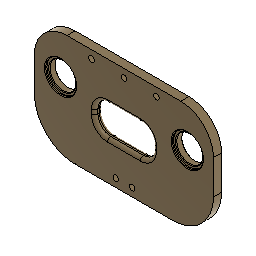
Outer Plate (Autodesk Fusion 360 design; units mm, degrees)
Autodesk Fusion 360 part; units mm, degrees
sketch "Sketch1" plane through (0, 58.6943, 0) normal (0, 1, 0) x (-1, 0, 0)
  line L0 (-161.4765, 498.7395) -> (-162.948, 497.802)
  line L1 (-162.948, 497.802) -> (-164.3322, 496.7399)
  line L2 (-164.3322, 496.7399) -> (-165.6186, 495.5611)
  line L3 (-165.6186, 495.5611) -> (-166.7974, 494.2748)
  line L4 (-166.7974, 494.2748) -> (-167.8595, 492.8905)
  line L5 (-167.8595, 492.8905) -> (-168.797, 491.419)
  line L6 (-168.797, 491.419) -> (-169.6026, 489.8714)
  line L7 (-169.6026, 489.8714) -> (-170.2703, 488.2594)
  line L8 (-170.2703, 488.2594) -> (-170.795, 486.5954)
  line L9 (-170.795, 486.5954) -> (-171.1726, 484.892)
  line L10 (-171.1726, 484.892) -> (-171.4004, 483.1621)
  line L11 (-171.4004, 483.1621) -> (-171.4765, 481.419)
  line L12 (-171.4765, 481.419) -> (-171.4765, 460.419)
  line L13 (-171.4765, 460.419) -> (-171.3994, 458.4576)
  line L14 (-171.3994, 458.4576) -> (-171.1687, 456.5082)
  line L15 (-171.1687, 456.5082) -> (-170.7857, 454.5829)
  line L16 (-170.7857, 454.5829) -> (-170.2529, 452.6936)
  line L17 (-170.2529, 452.6936) -> (-169.5735, 450.8519)
  line L18 (-169.5735, 450.8519) -> (-168.7516, 449.0692)
  line L19 (-168.7516, 449.0692) -> (-167.7925, 447.3565)
  line L20 (-167.7925, 447.3565) -> (-166.7019, 445.7244)
  line L21 (-166.7019, 445.7244) -> (-165.4866, 444.1828)
  line L22 (-165.4866, 444.1828) -> (-164.1541, 442.7413)
  line L23 (-164.1541, 442.7413) -> (-162.7127, 441.4089)
  line L24 (-162.7127, 441.4089) -> (-161.1711, 440.1936)
  line L25 (-161.1711, 440.1936) -> (-159.5389, 439.103)
  line L26 (-159.5389, 439.103) -> (-157.8262, 438.1439)
  line L27 (-157.8262, 438.1439) -> (-156.0436, 437.322)
  line L28 (-156.0436, 437.322) -> (-154.2019, 436.6426)
  line L29 (-154.2019, 436.6426) -> (-152.3126, 436.1098)
  line L30 (-152.3126, 436.1098) -> (-150.3873, 435.7268)
  line L31 (-150.3873, 435.7268) -> (-148.4379, 435.4961)
  line L32 (-148.4379, 435.4961) -> (-146.4765, 435.419)
  line L33 (-146.4765, 435.419) -> (-86.4765, 435.419)
  line L34 (-86.4765, 435.419) -> (-84.515, 435.4961)
  line L35 (-84.515, 435.4961) -> (-82.5656, 435.7268)
  line L36 (-82.5656, 435.7268) -> (-80.6403, 436.1098)
  line L37 (-80.6403, 436.1098) -> (-78.751, 436.6426)
  line L38 (-78.751, 436.6426) -> (-76.9094, 437.322)
  line L39 (-76.9094, 437.322) -> (-75.1267, 438.1439)
  line L40 (-75.1267, 438.1439) -> (-73.414, 439.103)
  line L41 (-73.414, 439.103) -> (-71.7818, 440.1936)
  line L42 (-71.7818, 440.1936) -> (-70.2403, 441.4089)
  line L43 (-70.2403, 441.4089) -> (-68.7988, 442.7413)
  line L44 (-68.7988, 442.7413) -> (-67.4663, 444.1828)
  line L45 (-67.4663, 444.1828) -> (-66.251, 445.7244)
  line L46 (-66.251, 445.7244) -> (-65.1605, 447.3565)
  line L47 (-65.1605, 447.3565) -> (-64.2013, 449.0692)
  line L48 (-64.2013, 449.0692) -> (-63.3795, 450.8519)
  line L49 (-63.3795, 450.8519) -> (-62.7, 452.6936)
  line L50 (-62.7, 452.6936) -> (-62.1672, 454.5829)
  line L51 (-62.1672, 454.5829) -> (-61.7843, 456.5082)
  line L52 (-61.7843, 456.5082) -> (-61.5535, 458.4576)
  line L53 (-61.5535, 458.4576) -> (-61.4765, 460.419)
  line L54 (-61.4765, 460.419) -> (-61.4765, 481.419)
  line L55 (-61.4765, 481.419) -> (-61.5526, 483.1621)
  line L56 (-61.5526, 483.1621) -> (-61.7803, 484.892)
  line L57 (-61.7803, 484.892) -> (-62.1579, 486.5954)
  line L58 (-62.1579, 486.5954) -> (-62.6826, 488.2594)
  line L59 (-62.6826, 488.2594) -> (-63.3503, 489.8714)
  line L60 (-63.3503, 489.8714) -> (-64.1559, 491.419)
  line L61 (-64.1559, 491.419) -> (-65.0934, 492.8905)
  line L62 (-65.0934, 492.8905) -> (-66.1556, 494.2748)
  line L63 (-66.1556, 494.2748) -> (-67.3343, 495.5611)
  line L64 (-67.3343, 495.5611) -> (-68.6207, 496.7399)
  line L65 (-68.6207, 496.7399) -> (-70.0049, 497.802)
  line L66 (-70.0049, 497.802) -> (-71.4765, 498.7395)
  line L67 (-71.4765, 498.7395) -> (-73.0241, 499.5452)
  line L68 (-73.0241, 499.5452) -> (-74.6361, 500.2129)
  line L69 (-74.6361, 500.2129) -> (-76.3001, 500.7375)
  line L70 (-76.3001, 500.7375) -> (-78.0035, 501.1151)
  line L71 (-78.0035, 501.1151) -> (-79.7333, 501.3429)
  line L72 (-79.7333, 501.3429) -> (-81.4765, 501.419)
  line L73 (-81.4765, 501.419) -> (-151.4765, 501.419)
  line L74 (-151.4765, 501.419) -> (-153.2196, 501.3429)
  line L75 (-153.2196, 501.3429) -> (-154.9494, 501.1151)
  line L76 (-154.9494, 501.1151) -> (-156.6528, 500.7375)
  line L77 (-156.6528, 500.7375) -> (-158.3169, 500.2129)
  line L78 (-158.3169, 500.2129) -> (-159.9288, 499.5452)
  line L79 (-159.9288, 499.5452) -> (-161.4765, 498.7395)
  line L80 (-124.4561, 440.0705) -> (-124.4561, 440.767)
  line L81 (-124.4561, 440.767) -> (-124.2954, 441.4448)
  line L82 (-124.2954, 441.4448) -> (-123.9828, 442.0672)
  line L83 (-123.9828, 442.0672) -> (-123.5351, 442.6007)
  line L84 (-123.5351, 442.6007) -> (-122.9765, 443.0167)
  line L85 (-122.9765, 443.0167) -> (-122.3369, 443.2925)
  line L86 (-122.3369, 443.2925) -> (-121.651, 443.4135)
  line L87 (-121.651, 443.4135) -> (-120.9557, 443.373)
  line L88 (-120.9557, 443.373) -> (-120.2884, 443.1732)
  line L89 (-120.2884, 443.1732) -> (-119.6852, 442.825)
  line L90 (-119.6852, 442.825) -> (-119.1786, 442.347)
  line L91 (-119.1786, 442.347) -> (-118.7959, 441.7651)
  line L92 (-118.7959, 441.7651) -> (-118.5577, 441.1106)
  line L93 (-118.5577, 441.1106) -> (-118.4768, 440.4188)
  line L94 (-118.4768, 440.4188) -> (-118.5577, 439.727)
  line L95 (-118.5577, 439.727) -> (-118.7959, 439.0725)
  line L96 (-118.7959, 439.0725) -> (-119.1786, 438.4906)
  line L97 (-119.1786, 438.4906) -> (-119.6852, 438.0126)
  line L98 (-119.6852, 438.0126) -> (-120.2884, 437.6643)
  line L99 (-120.2884, 437.6643) -> (-120.9557, 437.4646)
  line L100 (-120.9557, 437.4646) -> (-121.651, 437.4241)
  line L101 (-121.651, 437.4241) -> (-122.3369, 437.545)
  line L102 (-122.3369, 437.545) -> (-122.9765, 437.8209)
  line L103 (-122.9765, 437.8209) -> (-123.5351, 438.2369)
  line L104 (-123.5351, 438.2369) -> (-123.9828, 438.7704)
  line L105 (-123.9828, 438.7704) -> (-124.2954, 439.3928)
  line L106 (-124.2954, 439.3928) -> (-124.4561, 440.0705)
  line L107 (-90.9566, 487.2028) -> (-90.3766, 487.4647)
  line L108 (-90.3766, 487.4647) -> (-89.75, 487.5755)
  line L109 (-89.75, 487.5755) -> (-89.1154, 487.5283)
  line L110 (-89.1154, 487.5283) -> (-88.5121, 487.326)
  line L111 (-88.5121, 487.326) -> (-83.3137, 484.827)
  line L112 (-83.3137, 484.827) -> (-82.2929, 493.5729)
  line L113 (-82.2929, 493.5729) -> (-82.1336, 493.5729)
  line L114 (-82.1336, 493.5729) -> (-82.0349, 494.419)
  line L115 (-82.0349, 494.419) -> (-80.1169, 494.419)
  line L116 (-80.1169, 494.419) -> (-80.1158, 494.4247)
  line L117 (-80.1158, 494.4247) -> (-79.9215, 495.053)
  line L118 (-79.9215, 495.053) -> (-79.5884, 495.6199)
  line L119 (-79.5884, 495.6199) -> (-79.1342, 496.0954)
  line L120 (-79.1342, 496.0954) -> (-78.5831, 496.4542)
  line L121 (-78.5831, 496.4542) -> (-77.9645, 496.6771)
  line L122 (-77.9645, 496.6771) -> (-77.3112, 496.7523)
  line L123 (-77.3112, 496.7523) -> (-76.6581, 496.6758)
  line L124 (-76.6581, 496.6758) -> (-76.04, 496.4516)
  line L125 (-76.04, 496.4516) -> (-75.4896, 496.0917)
  line L126 (-75.4896, 496.0917) -> (-75.0364, 495.6152)
  line L127 (-75.0364, 495.6152) -> (-74.7044, 495.0476)
  line L128 (-74.7044, 495.0476) -> (-74.5114, 494.419)
  line L129 (-74.5114, 494.419) -> (-73.034, 494.419)
  line L130 (-73.034, 494.419) -> (-72.9352, 493.5729)
  line L131 (-72.9352, 493.5729) -> (-72.6609, 493.5729)
  line L132 (-72.6609, 493.5729) -> (-71.6401, 484.8274)
  line L133 (-71.6401, 484.8274) -> (-66.4424, 487.326)
  line L134 (-66.4424, 487.326) -> (-65.8391, 487.5283)
  line L135 (-65.8391, 487.5283) -> (-65.2045, 487.5755)
  line L136 (-65.2045, 487.5755) -> (-64.5779, 487.4647)
  line L137 (-64.5779, 487.4647) -> (-63.9979, 487.2028)
  line L138 (-63.9979, 487.2028) -> (-63.5005, 486.806)
  line L139 (-63.5005, 486.806) -> (-63.1163, 486.2987)
  line L140 (-63.1163, 486.2987) -> (-62.5715, 485.355)
  line L141 (-62.5715, 485.355) -> (-62.3346, 484.8044)
  line L142 (-62.3346, 484.8044) -> (-62.2323, 484.2138)
  line L143 (-62.2323, 484.2138) -> (-62.2701, 483.6156)
  line L144 (-62.2701, 483.6156) -> (-62.4459, 483.0425)
  line L145 (-62.4459, 483.0425) -> (-62.7502, 482.5261)
  line L146 (-62.7502, 482.5261) -> (-63.1661, 482.0945)
  line L147 (-63.1661, 482.0945) -> (-68.93, 477.3722)
  line L148 (-68.93, 477.3722) -> (-63.1661, 472.6498)
  line L149 (-63.1661, 472.6498) -> (-62.7502, 472.2182)
  line L150 (-62.7502, 472.2182) -> (-62.4459, 471.7018)
  line L151 (-62.4459, 471.7018) -> (-62.2701, 471.1287)
  line L152 (-62.2701, 471.1287) -> (-62.2323, 470.5305)
  line L153 (-62.2323, 470.5305) -> (-62.3346, 469.9399)
  line L154 (-62.3346, 469.9399) -> (-62.5715, 469.3893)
  line L155 (-62.5715, 469.3893) -> (-63.1163, 468.4456)
  line L156 (-63.1163, 468.4456) -> (-63.5005, 467.9383)
  line L157 (-63.5005, 467.9383) -> (-63.9979, 467.5415)
  line L158 (-63.9979, 467.5415) -> (-64.5779, 467.2796)
  line L159 (-64.5779, 467.2796) -> (-65.2045, 467.1688)
  line L160 (-65.2045, 467.1688) -> (-65.8391, 467.216)
  line L161 (-65.8391, 467.216) -> (-66.4424, 467.4183)
  line L162 (-66.4424, 467.4183) -> (-71.6506, 469.922)
  line L163 (-71.6506, 469.922) -> (-73.8018, 451.4907)
  line L164 (-73.8018, 451.4907) -> (-73.9694, 450.7417)
  line L165 (-73.9694, 450.7417) -> (-74.2878, 450.0434)
  line L166 (-74.2878, 450.0434) -> (-74.7435, 449.4259)
  line L167 (-74.7435, 449.4259) -> (-75.3168, 448.9156)
  line L168 (-75.3168, 448.9156) -> (-75.983, 448.5346)
  line L169 (-75.983, 448.5346) -> (-76.7135, 448.2992)
  line L170 (-76.7135, 448.2992) -> (-77.4769, 448.2196)
  line L171 (-77.4769, 448.2196) -> (-78.2402, 448.2992)
  line L172 (-78.2402, 448.2992) -> (-78.9707, 448.5346)
  line L173 (-78.9707, 448.5346) -> (-79.6369, 448.9156)
  line L174 (-79.6369, 448.9156) -> (-80.2102, 449.4259)
  line L175 (-80.2102, 449.4259) -> (-80.6659, 450.0434)
  line L176 (-80.6659, 450.0434) -> (-80.9844, 450.7417)
  line L177 (-80.9844, 450.7417) -> (-81.1519, 451.4907)
  line L178 (-81.1519, 451.4907) -> (-83.3277, 470.1324)
  line L179 (-83.3277, 470.1324) -> (-88.5987, 467.5986)
  line L180 (-88.5987, 467.5986) -> (-89.1549, 467.4121)
  line L181 (-89.1549, 467.4121) -> (-89.7399, 467.3686)
  line L182 (-89.7399, 467.3686) -> (-90.3176, 467.4707)
  line L183 (-90.3176, 467.4707) -> (-90.8523, 467.7121)
  line L184 (-90.8523, 467.7121) -> (-91.3108, 468.078)
  line L185 (-91.3108, 468.078) -> (-91.665, 468.5456)
  line L186 (-91.665, 468.5456) -> (-92.2102, 469.49)
  line L187 (-92.2102, 469.49) -> (-92.4286, 469.9976)
  line L188 (-92.4286, 469.9976) -> (-92.5229, 470.5421)
  line L189 (-92.5229, 470.5421) -> (-92.4881, 471.0935)
  line L190 (-92.4881, 471.0935) -> (-92.326, 471.6218)
  line L191 (-92.326, 471.6218) -> (-92.0455, 472.0979)
  line L192 (-92.0455, 472.0979) -> (-91.662, 472.4957)
  line L193 (-91.662, 472.4957) -> (-85.8673, 477.2434)
  line L194 (-85.8673, 477.2434) -> (-91.7884, 482.0945)
  line L195 (-91.7884, 482.0945) -> (-92.2044, 482.5261)
  line L196 (-92.2044, 482.5261) -> (-92.5086, 483.0425)
  line L197 (-92.5086, 483.0425) -> (-92.6845, 483.6156)
  line L198 (-92.6845, 483.6156) -> (-92.7222, 484.2138)
  line L199 (-92.7222, 484.2138) -> (-92.6199, 484.8044)
  line L200 (-92.6199, 484.8044) -> (-92.383, 485.355)
  line L201 (-92.383, 485.355) -> (-91.8382, 486.2987)
  line L202 (-91.8382, 486.2987) -> (-91.454, 486.806)
  line L203 (-91.454, 486.806) -> (-90.9566, 487.2028)
  line L204 (-97.3367, 499.2923) -> (-96.6509, 499.4133)
  line L205 (-96.6509, 499.4133) -> (-95.9555, 499.3728)
  line L206 (-95.9555, 499.3728) -> (-95.2883, 499.173)
  line L207 (-95.2883, 499.173) -> (-94.6852, 498.8248)
  line L208 (-94.6852, 498.8248) -> (-94.1785, 498.3468)
  line L209 (-94.1785, 498.3468) -> (-93.7958, 497.7649)
  line L210 (-93.7958, 497.7649) -> (-93.5576, 497.1104)
  line L211 (-93.5576, 497.1104) -> (-93.4768, 496.4187)
  line L212 (-93.4768, 496.4187) -> (-93.5576, 495.7269)
  line L213 (-93.5576, 495.7269) -> (-93.7958, 495.0724)
  line L214 (-93.7958, 495.0724) -> (-94.1785, 494.4905)
  line L215 (-94.1785, 494.4905) -> (-94.6852, 494.0126)
  line L216 (-94.6852, 494.0126) -> (-95.2883, 493.6643)
  line L217 (-95.2883, 493.6643) -> (-95.9555, 493.4646)
  line L218 (-95.9555, 493.4646) -> (-96.6509, 493.4241)
  line L219 (-96.6509, 493.4241) -> (-97.3367, 493.545)
  line L220 (-97.3367, 493.545) -> (-97.9763, 493.8209)
  line L221 (-97.9763, 493.8209) -> (-98.5349, 494.2368)
  line L222 (-98.5349, 494.2368) -> (-98.9826, 494.7703)
  line L223 (-98.9826, 494.7703) -> (-99.2952, 495.3927)
  line L224 (-99.2952, 495.3927) -> (-99.4558, 496.0704)
  line L225 (-99.4558, 496.0704) -> (-99.4558, 496.7669)
  line L226 (-99.4558, 496.7669) -> (-99.2952, 497.4446)
  line L227 (-99.2952, 497.4446) -> (-98.9826, 498.067)
  line L228 (-98.9826, 498.067) -> (-98.5349, 498.6006)
  line L229 (-98.5349, 498.6006) -> (-97.9763, 499.0165)
  line L230 (-97.9763, 499.0165) -> (-97.3367, 499.2923)
  line L231 (-108.4759, 440.4192) -> (-108.5568, 439.7273)
  line L232 (-108.5568, 439.7273) -> (-108.7951, 439.0726)
  line L233 (-108.7951, 439.0726) -> (-109.1779, 438.4906)
  line L234 (-109.1779, 438.4906) -> (-109.6846, 438.0126)
  line L235 (-109.6846, 438.0126) -> (-110.2879, 437.6642)
  line L236 (-110.2879, 437.6642) -> (-110.9552, 437.4645)
  line L237 (-110.9552, 437.4645) -> (-111.6507, 437.424)
  line L238 (-111.6507, 437.424) -> (-112.3367, 437.5449)
  line L239 (-112.3367, 437.5449) -> (-112.9764, 437.8208)
  line L240 (-112.9764, 437.8208) -> (-113.5351, 438.2369)
  line L241 (-113.5351, 438.2369) -> (-113.9829, 438.7705)
  line L242 (-113.9829, 438.7705) -> (-114.2956, 439.393)
  line L243 (-114.2956, 439.393) -> (-114.4562, 440.0709)
  line L244 (-114.4562, 440.0709) -> (-114.4562, 440.7675)
  line L245 (-114.4562, 440.7675) -> (-114.2956, 441.4453)
  line L246 (-114.2956, 441.4453) -> (-113.9829, 442.0678)
  line L247 (-113.9829, 442.0678) -> (-113.5351, 442.6015)
  line L248 (-113.5351, 442.6015) -> (-112.9764, 443.0175)
  line L249 (-112.9764, 443.0175) -> (-112.3367, 443.2934)
  line L250 (-112.3367, 443.2934) -> (-111.6507, 443.4144)
  line L251 (-111.6507, 443.4144) -> (-110.9552, 443.3739)
  line L252 (-110.9552, 443.3739) -> (-110.2879, 443.1741)
  line L253 (-110.2879, 443.1741) -> (-109.6846, 442.8257)
  line L254 (-109.6846, 442.8257) -> (-109.1779, 442.3477)
  line L255 (-109.1779, 442.3477) -> (-108.7951, 441.7657)
  line L256 (-108.7951, 441.7657) -> (-108.5568, 441.1111)
  line L257 (-108.5568, 441.1111) -> (-108.4759, 440.4192)
  line L258 (-133.9616, 488.0502) -> (-133.1077, 488.9041)
  line L259 (-133.1077, 488.9041) -> (-132.1571, 489.6488)
  line L260 (-132.1571, 489.6488) -> (-131.1237, 490.2736)
  line L261 (-131.1237, 490.2736) -> (-130.0225, 490.7692)
  line L262 (-130.0225, 490.7692) -> (-128.8696, 491.1284)
  line L263 (-128.8696, 491.1284) -> (-127.6818, 491.3461)
  line L264 (-127.6818, 491.3461) -> (-126.4765, 491.419)
  line L265 (-126.4765, 491.419) -> (-106.4765, 491.419)
  line L266 (-106.4765, 491.419) -> (-105.2711, 491.3461)
  line L267 (-105.2711, 491.3461) -> (-104.0833, 491.1284)
  line L268 (-104.0833, 491.1284) -> (-102.9304, 490.7692)
  line L269 (-102.9304, 490.7692) -> (-101.8292, 490.2736)
  line L270 (-101.8292, 490.2736) -> (-100.7958, 489.6488)
  line L271 (-100.7958, 489.6488) -> (-99.8452, 488.9041)
  line L272 (-99.8452, 488.9041) -> (-98.9914, 488.0502)
  line L273 (-98.9914, 488.0502) -> (-98.2466, 487.0996)
  line L274 (-98.2466, 487.0996) -> (-97.6219, 486.0662)
  line L275 (-97.6219, 486.0662) -> (-97.1263, 484.9651)
  line L276 (-97.1263, 484.9651) -> (-96.767, 483.8122)
  line L277 (-96.767, 483.8122) -> (-96.5494, 482.6244)
  line L278 (-96.5494, 482.6244) -> (-96.4765, 481.419)
  line L279 (-96.4765, 481.419) -> (-96.4765, 455.419)
  line L280 (-96.4765, 455.419) -> (-96.5494, 454.2137)
  line L281 (-96.5494, 454.2137) -> (-96.767, 453.0259)
  line L282 (-96.767, 453.0259) -> (-97.1263, 451.873)
  line L283 (-97.1263, 451.873) -> (-97.6219, 450.7718)
  line L284 (-97.6219, 450.7718) -> (-98.2466, 449.7384)
  line L285 (-98.2466, 449.7384) -> (-98.9914, 448.7878)
  line L286 (-98.9914, 448.7878) -> (-99.8452, 447.9339)
  line L287 (-99.8452, 447.9339) -> (-100.7958, 447.1892)
  line L288 (-100.7958, 447.1892) -> (-101.8292, 446.5645)
  line L289 (-101.8292, 446.5645) -> (-102.9304, 446.0689)
  line L290 (-102.9304, 446.0689) -> (-104.0833, 445.7096)
  line L291 (-104.0833, 445.7096) -> (-105.2711, 445.4919)
  line L292 (-105.2711, 445.4919) -> (-106.4765, 445.419)
  line L293 (-106.4765, 445.419) -> (-126.4765, 445.419)
  line L294 (-126.4765, 445.419) -> (-127.6818, 445.4919)
  line L295 (-127.6818, 445.4919) -> (-128.8696, 445.7096)
  line L296 (-128.8696, 445.7096) -> (-130.0225, 446.0689)
  line L297 (-130.0225, 446.0689) -> (-131.1237, 446.5645)
  line L298 (-131.1237, 446.5645) -> (-132.1571, 447.1892)
  line L299 (-132.1571, 447.1892) -> (-133.1077, 447.9339)
  line L300 (-133.1077, 447.9339) -> (-133.9616, 448.7878)
  line L301 (-133.9616, 448.7878) -> (-134.7063, 449.7384)
  line L302 (-134.7063, 449.7384) -> (-135.331, 450.7718)
  line L303 (-135.331, 450.7718) -> (-135.8266, 451.873)
  line L304 (-135.8266, 451.873) -> (-136.1859, 453.0259)
  line L305 (-136.1859, 453.0259) -> (-136.4036, 454.2137)
  line L306 (-136.4036, 454.2137) -> (-136.4765, 455.419)
  line L307 (-136.4765, 455.419) -> (-136.4765, 481.419)
  line L308 (-136.4765, 481.419) -> (-136.4036, 482.6244)
  line L309 (-136.4036, 482.6244) -> (-136.1859, 483.8122)
  line L310 (-136.1859, 483.8122) -> (-135.8266, 484.9651)
  line L311 (-135.8266, 484.9651) -> (-135.331, 486.0662)
  line L312 (-135.331, 486.0662) -> (-134.7063, 487.0996)
  line L313 (-134.7063, 487.0996) -> (-133.9616, 488.0502)
  line L314 (-139.2957, 497.4455) -> (-138.983, 498.0681)
  line L315 (-138.983, 498.0681) -> (-138.5352, 498.6017)
  line L316 (-138.5352, 498.6017) -> (-137.9765, 499.0177)
  line L317 (-137.9765, 499.0177) -> (-137.3368, 499.2936)
  line L318 (-137.3368, 499.2936) -> (-136.6507, 499.4146)
  line L319 (-136.6507, 499.4146) -> (-135.9553, 499.3741)
  line L320 (-135.9553, 499.3741) -> (-135.2879, 499.1743)
  line L321 (-135.2879, 499.1743) -> (-134.6846, 498.826)
  line L322 (-134.6846, 498.826) -> (-134.1779, 498.3479)
  line L323 (-134.1779, 498.3479) -> (-133.795, 497.7659)
  line L324 (-133.795, 497.7659) -> (-133.5568, 497.1113)
  line L325 (-133.5568, 497.1113) -> (-133.4759, 496.4193)
  line L326 (-133.4759, 496.4193) -> (-133.5568, 495.7274)
  line L327 (-133.5568, 495.7274) -> (-133.795, 495.0728)
  line L328 (-133.795, 495.0728) -> (-134.1779, 494.4907)
  line L329 (-134.1779, 494.4907) -> (-134.6846, 494.0127)
  line L330 (-134.6846, 494.0127) -> (-135.2879, 493.6643)
  line L331 (-135.2879, 493.6643) -> (-135.9553, 493.4645)
  line L332 (-135.9553, 493.4645) -> (-136.6507, 493.424)
  line L333 (-136.6507, 493.424) -> (-137.3368, 493.545)
  line L334 (-137.3368, 493.545) -> (-137.9765, 493.821)
  line L335 (-137.9765, 493.821) -> (-138.5352, 494.2369)
  line L336 (-138.5352, 494.2369) -> (-138.983, 494.7706)
  line L337 (-138.983, 494.7706) -> (-139.2957, 495.3932)
  line L338 (-139.2957, 495.3932) -> (-139.4563, 496.071)
  line L339 (-139.4563, 496.071) -> (-139.4563, 496.7676)
  line L340 (-139.4563, 496.7676) -> (-139.2957, 497.4455)
  line L341 (-157.4607, 494.419) -> (-157.4597, 494.4247)
  line L342 (-157.4597, 494.4247) -> (-157.2654, 495.0529)
  line L343 (-157.2654, 495.0529) -> (-156.9322, 495.6198)
  line L344 (-156.9322, 495.6198) -> (-156.478, 496.0954)
  line L345 (-156.478, 496.0954) -> (-155.927, 496.4541)
  line L346 (-155.927, 496.4541) -> (-155.3083, 496.677)
  line L347 (-155.3083, 496.677) -> (-154.6551, 496.7522)
  line L348 (-154.6551, 496.7522) -> (-154.002, 496.6757)
  line L349 (-154.002, 496.6757) -> (-153.3839, 496.4515)
  line L350 (-153.3839, 496.4515) -> (-152.8335, 496.0917)
  line L351 (-152.8335, 496.0917) -> (-152.3803, 495.6152)
  line L352 (-152.3803, 495.6152) -> (-152.0483, 495.0476)
  line L353 (-152.0483, 495.0476) -> (-151.8553, 494.419)
  line L354 (-151.8553, 494.419) -> (-151.034, 494.419)
  line L355 (-151.034, 494.419) -> (-150.9352, 493.5729)
  line L356 (-150.9352, 493.5729) -> (-150.0047, 493.5729)
  line L357 (-150.0047, 493.5729) -> (-148.984, 484.8273)
  line L358 (-148.984, 484.8273) -> (-143.7863, 487.326)
  line L359 (-143.7863, 487.326) -> (-143.1829, 487.5282)
  line L360 (-143.1829, 487.5282) -> (-142.5484, 487.5754)
  line L361 (-142.5484, 487.5754) -> (-141.9217, 487.4647)
  line L362 (-141.9217, 487.4647) -> (-141.3418, 487.2028)
  line L363 (-141.3418, 487.2028) -> (-140.8444, 486.8059)
  line L364 (-140.8444, 486.8059) -> (-140.4602, 486.2986)
  line L365 (-140.4602, 486.2986) -> (-139.9153, 485.355)
  line L366 (-139.9153, 485.355) -> (-139.6785, 484.8043)
  line L367 (-139.6785, 484.8043) -> (-139.5761, 484.2137)
  line L368 (-139.5761, 484.2137) -> (-139.6139, 483.6155)
  line L369 (-139.6139, 483.6155) -> (-139.7898, 483.0425)
  line L370 (-139.7898, 483.0425) -> (-140.094, 482.526)
  line L371 (-140.094, 482.526) -> (-140.51, 482.0945)
  line L372 (-140.51, 482.0945) -> (-146.2739, 477.3721)
  line L373 (-146.2739, 477.3721) -> (-140.51, 472.6497)
  line L374 (-140.51, 472.6497) -> (-140.094, 472.2182)
  line L375 (-140.094, 472.2182) -> (-139.7898, 471.7017)
  line L376 (-139.7898, 471.7017) -> (-139.6139, 471.1287)
  line L377 (-139.6139, 471.1287) -> (-139.5761, 470.5305)
  line L378 (-139.5761, 470.5305) -> (-139.6785, 469.9399)
  line L379 (-139.6785, 469.9399) -> (-139.9153, 469.3893)
  line L380 (-139.9153, 469.3893) -> (-140.4602, 468.4456)
  line L381 (-140.4602, 468.4456) -> (-140.8444, 467.9383)
  line L382 (-140.8444, 467.9383) -> (-141.3418, 467.5414)
  line L383 (-141.3418, 467.5414) -> (-141.9217, 467.2795)
  line L384 (-141.9217, 467.2795) -> (-142.5484, 467.1687)
  line L385 (-142.5484, 467.1687) -> (-143.1829, 467.216)
  line L386 (-143.1829, 467.216) -> (-143.7863, 467.4182)
  line L387 (-143.7863, 467.4182) -> (-148.9945, 469.9219)
  line L388 (-148.9945, 469.9219) -> (-151.1457, 451.4907)
  line L389 (-151.1457, 451.4907) -> (-151.3108, 450.749)
  line L390 (-151.3108, 450.749) -> (-151.624, 450.0566)
  line L391 (-151.624, 450.0566) -> (-152.072, 449.4429)
  line L392 (-152.072, 449.4429) -> (-152.6359, 448.9336)
  line L393 (-152.6359, 448.9336) -> (-153.292, 448.5502)
  line L394 (-153.292, 448.5502) -> (-154.0126, 448.309)
  line L395 (-154.0126, 448.309) -> (-154.7673, 448.2201)
  line L396 (-154.7673, 448.2201) -> (-155.5242, 448.2871)
  line L397 (-155.5242, 448.2871) -> (-156.2479, 448.3606)
  line L398 (-156.2479, 448.3606) -> (-156.9408, 448.5822)
  line L399 (-156.9408, 448.5822) -> (-157.573, 448.9421)
  line L400 (-157.573, 448.9421) -> (-158.1171, 449.425)
  line L401 (-158.1171, 449.425) -> (-158.5496, 450.0099)
  line L402 (-158.5496, 450.0099) -> (-158.8519, 450.6715)
  line L403 (-158.8519, 450.6715) -> (-159.0108, 451.3814)
  line L404 (-159.0108, 451.3814) -> (-161.1713, 469.8922)
  line L405 (-161.1713, 469.8922) -> (-165.9426, 467.5985)
  line L406 (-165.9426, 467.5985) -> (-166.4988, 467.412)
  line L407 (-166.4988, 467.412) -> (-167.0838, 467.3685)
  line L408 (-167.0838, 467.3685) -> (-167.6615, 467.4706)
  line L409 (-167.6615, 467.4706) -> (-168.1961, 467.7121)
  line L410 (-168.1961, 467.7121) -> (-168.6547, 468.0779)
  line L411 (-168.6547, 468.0779) -> (-169.0089, 468.5456)
  line L412 (-169.0089, 468.5456) -> (-169.5541, 469.4899)
  line L413 (-169.5541, 469.4899) -> (-169.7724, 469.9975)
  line L414 (-169.7724, 469.9975) -> (-169.8668, 470.542)
  line L415 (-169.8668, 470.542) -> (-169.8319, 471.0935)
  line L416 (-169.8319, 471.0935) -> (-169.6698, 471.6217)
  line L417 (-169.6698, 471.6217) -> (-169.3894, 472.0978)
  line L418 (-169.3894, 472.0978) -> (-169.0059, 472.4956)
  line L419 (-169.0059, 472.4956) -> (-163.2111, 477.2433)
  line L420 (-163.2111, 477.2433) -> (-169.1322, 482.0945)
  line L421 (-169.1322, 482.0945) -> (-169.5482, 482.526)
  line L422 (-169.5482, 482.526) -> (-169.8525, 483.0425)
  line L423 (-169.8525, 483.0425) -> (-170.0283, 483.6155)
  line L424 (-170.0283, 483.6155) -> (-170.0661, 484.2137)
  line L425 (-170.0661, 484.2137) -> (-169.9637, 484.8043)
  line L426 (-169.9637, 484.8043) -> (-169.7269, 485.355)
  line L427 (-169.7269, 485.355) -> (-169.1821, 486.2986)
  line L428 (-169.1821, 486.2986) -> (-168.7979, 486.8059)
  line L429 (-168.7979, 486.8059) -> (-168.3004, 487.2028)
  line L430 (-168.3004, 487.2028) -> (-167.7205, 487.4647)
  line L431 (-167.7205, 487.4647) -> (-167.0939, 487.5754)
  line L432 (-167.0939, 487.5754) -> (-166.4593, 487.5282)
  line L433 (-166.4593, 487.5282) -> (-165.856, 487.326)
  line L434 (-165.856, 487.326) -> (-161.128, 485.0531)
  line L435 (-161.128, 485.0531) -> (-160.0349, 494.419)
  line L436 (-160.0349, 494.419) -> (-157.4607, 494.419)
  line L437 (-73.414, 439.103) -> (-71.7818, 440.1936)
  line L438 (-71.7818, 440.1936) -> (-70.2403, 441.4089)
  line L439 (-70.2403, 441.4089) -> (-68.7988, 442.7413)
  line L440 (-68.7988, 442.7413) -> (-67.4663, 444.1828)
  line L441 (-67.4663, 444.1828) -> (-66.251, 445.7244)
  line L442 (-66.251, 445.7244) -> (-65.1605, 447.3565)
  line L443 (-65.1605, 447.3565) -> (-64.2013, 449.0692)
  line L444 (-64.2013, 449.0692) -> (-63.3795, 450.8519)
  line L445 (-63.3795, 450.8519) -> (-62.7, 452.6936)
  line L446 (-62.7, 452.6936) -> (-62.1672, 454.5829)
  line L447 (-62.1672, 454.5829) -> (-61.7843, 456.5082)
  line L448 (-61.7843, 456.5082) -> (-61.5535, 458.4576)
  line L449 (-61.5535, 458.4576) -> (-61.4765, 460.419)
  line L450 (-61.4765, 460.419) -> (-61.4765, 481.419)
  line L451 (-61.4765, 481.419) -> (-61.5526, 483.1621)
  line L452 (-61.5526, 483.1621) -> (-61.7803, 484.892)
  line L453 (-61.7803, 484.892) -> (-62.1579, 486.5954)
  line L454 (-62.1579, 486.5954) -> (-62.6826, 488.2594)
  line L455 (-62.6826, 488.2594) -> (-63.3503, 489.8714)
  line L456 (-63.3503, 489.8714) -> (-64.1559, 491.419)
  line L457 (-64.1559, 491.419) -> (-65.0934, 492.8905)
  line L458 (-65.0934, 492.8905) -> (-66.1556, 494.2748)
  line L459 (-66.1556, 494.2748) -> (-67.3343, 495.5611)
  line L460 (-67.3343, 495.5611) -> (-68.6207, 496.7399)
  line L461 (-68.6207, 496.7399) -> (-70.0049, 497.802)
  line L462 (-70.0049, 497.802) -> (-71.4765, 498.7395)
  line L463 (-71.4765, 498.7395) -> (-73.0241, 499.5452)
  line L464 (-73.0241, 499.5452) -> (-74.6361, 500.2129)
  line L465 (-74.6361, 500.2129) -> (-76.3001, 500.7375)
  line L466 (-76.3001, 500.7375) -> (-78.0035, 501.1151)
  line L467 (-78.0035, 501.1151) -> (-79.7333, 501.3429)
  line L468 (-79.7333, 501.3429) -> (-81.4765, 501.419)
  line L469 (-81.4765, 501.419) -> (-151.4765, 501.419)
  line L470 (-151.4765, 501.419) -> (-153.2196, 501.3429)
  line L471 (-153.2196, 501.3429) -> (-154.9494, 501.1151)
  line L472 (-154.9494, 501.1151) -> (-156.6528, 500.7375)
  line L473 (-156.6528, 500.7375) -> (-158.3169, 500.2129)
  line L474 (-158.3169, 500.2129) -> (-159.9288, 499.5452)
  line L475 (-159.9288, 499.5452) -> (-161.4765, 498.7395)
  line L476 (-161.4765, 498.7395) -> (-162.948, 497.802)
  line L477 (-162.948, 497.802) -> (-164.3322, 496.7399)
  line L478 (-164.3322, 496.7399) -> (-165.6186, 495.5611)
  line L479 (-165.6186, 495.5611) -> (-166.7974, 494.2748)
  line L480 (-166.7974, 494.2748) -> (-167.8595, 492.8905)
  line L481 (-167.8595, 492.8905) -> (-168.797, 491.419)
  line L482 (-168.797, 491.419) -> (-169.6026, 489.8714)
  line L483 (-169.6026, 489.8714) -> (-170.2703, 488.2594)
  line L484 (-170.2703, 488.2594) -> (-170.795, 486.5954)
  line L485 (-170.795, 486.5954) -> (-171.1726, 484.892)
  line L486 (-171.1726, 484.892) -> (-171.4004, 483.1621)
  line L487 (-171.4004, 483.1621) -> (-171.4765, 481.419)
  line L488 (-171.4765, 481.419) -> (-171.4765, 460.419)
  line L489 (-171.4765, 460.419) -> (-171.3994, 458.4576)
  line L490 (-171.3994, 458.4576) -> (-171.1687, 456.5082)
  line L491 (-171.1687, 456.5082) -> (-170.7857, 454.5829)
  line L492 (-170.7857, 454.5829) -> (-170.2529, 452.6936)
  line L493 (-170.2529, 452.6936) -> (-169.5735, 450.8519)
  line L494 (-169.5735, 450.8519) -> (-168.7516, 449.0692)
  line L495 (-168.7516, 449.0692) -> (-167.7925, 447.3565)
  line L496 (-167.7925, 447.3565) -> (-166.7019, 445.7244)
  line L497 (-166.7019, 445.7244) -> (-165.4866, 444.1828)
  line L498 (-165.4866, 444.1828) -> (-164.1541, 442.7413)
  line L499 (-164.1541, 442.7413) -> (-162.7127, 441.4089)
  line L500 (-162.7127, 441.4089) -> (-161.1711, 440.1936)
  line L501 (-161.1711, 440.1936) -> (-159.5389, 439.103)
  line L502 (-159.5389, 439.103) -> (-157.8262, 438.1439)
  line L503 (-157.8262, 438.1439) -> (-156.0436, 437.322)
  line L504 (-156.0436, 437.322) -> (-154.2019, 436.6426)
  line L505 (-154.2019, 436.6426) -> (-152.3126, 436.1098)
  line L506 (-152.3126, 436.1098) -> (-150.3873, 435.7268)
  line L507 (-150.3873, 435.7268) -> (-148.4379, 435.4961)
  line L508 (-148.4379, 435.4961) -> (-146.4765, 435.419)
  line L509 (-146.4765, 435.419) -> (-86.4765, 435.419)
  line L510 (-86.4765, 435.419) -> (-84.515, 435.4961)
  line L511 (-84.515, 435.4961) -> (-82.5656, 435.7268)
  line L512 (-82.5656, 435.7268) -> (-80.6403, 436.1098)
  line L513 (-80.6403, 436.1098) -> (-78.751, 436.6426)
  line L514 (-78.751, 436.6426) -> (-76.9094, 437.322)
  line L515 (-76.9094, 437.322) -> (-75.1267, 438.1439)
  line L516 (-75.1267, 438.1439) -> (-73.414, 439.103)
  line L517 (-173.3125, 477.419) -> (-58.5356, 477.419) construction
  line L518 (-168.4954, 496.419) -> (-64.6373, 496.419) construction
  line L519 (-171.0003, 440.419) -> (-59.9486, 440.419) construction
  line L520 (-77.4765, 504.795) -> (-77.4765, 432.0043) construction
  line L521 (-155.4765, 503.6469) -> (-155.4765, 428.4834) construction
  line L522 (-116.4765, 501.419) -> (-116.4765, 435.419) construction
  line L523 (-121.4765, 453.8028) -> (-121.4765, 421.8293) construction
  line L524 (-111.4765, 453.5235) -> (-111.4765, 425.7387) construction
  line L525 (-96.4765, 506.1611) -> (-96.4765, 488.6249) construction
  line L526 (-136.4765, 507.4177) -> (-136.4765, 490.3838) construction
  point P0 (-155.4765, 477.419)
  point P1 (-77.4765, 477.419)
  point P2 (-96.4765, 496.419)
  point P3 (-136.4765, 496.419)
  point P4 (-121.4765, 440.419)
  point P5 (-111.4765, 440.419)
  point P6 (-116.5663, 496.419)
  dimension "d1" = 0
  dimension "d2" = 5
  dimension "d3" = 5
  dimension "d4" = 24
  dimension "d5" = 78
  dimension "d6" = 39
  dimension "d30" = 66
  dimension "d31" = 110
  dimension "d32" = 10
  dimension "d33" = 5
  dimension "d34" = 40
  dimension "d35" = 20
  constraint horizontal L517
  constraint horizontal L518
  constraint horizontal L519
  constraint parallel L488 L520
  constraint perpendicular L519 L521
  constraint midpoint L469 L522.start
  constraint midpoint L509 L522.end
  constraint parallel L80 L523
  constraint perpendicular L509 L524
  constraint vertical L525
  constraint perpendicular L518 L526
  constraint coincident L517 P0
  constraint coincident L521 P0
  constraint coincident L517 P1
  constraint coincident L520 P1
  constraint coincident L518 P2
  constraint coincident L525 P2
  constraint coincident L518 P3
  constraint coincident L526 P3
  constraint coincident L523 P4
  constraint coincident L519 P4
  constraint coincident L519 P5
  constraint coincident L524 P5
  constraint midpoint L518 P6
  measures "d2" distance of L469 L518
  measures "d3" distance of L509 L519
  measures "d4" distance of L469 L517
  measures "d5" distance of L520 L521
  measures "d6" distance of L521 L522
  measures "d30" distance of L469 L509
  measures "d31" distance of L450 L488
  measures "d32" distance of L523 L524
  measures "d33" distance of L522 L523
  measures "d34" distance of L525 L526
  measures "d35" distance of L522 L525
sketch "Sketch2" plane through (267.0969, 53.6943, 58.2152) normal (0, -1, 0) x (1, 0, 0)
  line L0 (-185.6204, 443.2039) -> (-115.6204, 443.2039)
  line L1 (-115.6204, 443.2039) -> (-185.6204, 443.2039)
  line L2 (-95.6204, 423.2039) -> (-95.6204, 402.2039)
  line L3 (-205.6204, 423.2039) -> (-205.6204, 402.2039)
  line L4 (-205.6204, 423.2039) -> (-205.6204, 402.2039)
  line L5 (-95.6204, 402.2039) -> (-95.6204, 423.2039)
  arc A0 (-185.6204, 443.2039) -> (-205.6204, 423.2039) centre (-185.6204, 423.2039) ccw
  arc A1 (-95.6204, 423.2039) -> (-115.6204, 443.2039) centre (-115.6204, 423.2039) ccw
  arc A2 (-205.6204, 402.2039) -> (-180.6204, 377.2039) centre (-180.6204, 402.2039) ccw
  arc A3 (-120.6204, 377.2039) -> (-95.6204, 402.2039) centre (-120.6204, 402.2039) ccw
  line L6 (-180.6204, 377.2039) -> (-120.6204, 377.2039)
  dimension "d88" = 20
  dimension "d89" = 25
  constraint collinear L0 L1
  constraint vertical L2
  constraint collinear L3 L4
  constraint collinear L2 L5
  constraint tangent L0 A0
  constraint tangent L3 A0
  constraint tangent L0 A1
  constraint tangent L2 A1
  constraint equal A0 A1
  constraint tangent L3 A2
  constraint tangent L2 A3
  constraint equal A2 A3
  constraint tangent A2 L6
  measures "d88" radius of A0
  measures "d89" radius of A2
extrude "Extrude8" add sketch "Sketch2" against normal blind 5
hole "Hole3" at (77.4765, 58.6943, 477.419) at (155.4765, 58.6943, 477.419) direction (0, -1, 0) diameter 16 depth 10 tip angle 118
hole "Hole4" at (136.4765, 58.6943, 496.419) at (116.5663, 58.6943, 496.419) at (96.4765, 58.6943, 496.419) at (121.4765, 58.6943, 440.419) at (111.4765, 58.6943, 440.419) direction (0, -1, 0) diameter 3.4 depth 5 tip angle 180
sketch "Sketch3" plane through (0, 58.6943, 0) normal (0, 1, 0) x (-1, 0, 0)
  circle A0 centre (-77.4765, 477.419) radius 8
  circle A1 centre (-155.4765, 477.419) radius 8
  line L0 (-146.4765, 435.419) -> (-86.4765, 435.419)
  arc A2 (-86.4765, 435.419) -> (-61.4765, 460.419) centre (-86.4765, 460.419) ccw
  line L1 (-61.4765, 460.419) -> (-61.4765, 481.419)
  arc A3 (-61.4765, 481.419) -> (-81.4765, 501.419) centre (-81.4765, 481.419) ccw
  line L2 (-81.4765, 501.419) -> (-151.4765, 501.419)
  arc A4 (-151.4765, 501.419) -> (-171.4765, 481.419) centre (-151.4765, 481.419) ccw
  line L3 (-171.4765, 481.419) -> (-171.4765, 460.419)
  arc A5 (-171.4765, 460.419) -> (-146.4765, 435.419) centre (-146.4765, 460.419) ccw
  line L4 (-147.4765, 491.719) -> (-85.4765, 491.719) construction
  line L5 (-85.4765, 491.719) -> (-85.4765, 445.119) construction
  line L6 (-85.4765, 445.119) -> (-147.4765, 445.119) construction
  line L7 (-147.4765, 445.119) -> (-147.4765, 491.719) construction
  arc A6 (-73.4765, 481.419) -> (-81.4765, 489.419) centre (-81.4765, 481.419) ccw
  line L8 (-81.4765, 489.419) -> (-151.4765, 489.419)
  arc A7 (-151.4765, 489.419) -> (-159.4765, 481.419) centre (-151.4765, 481.419) ccw
  line L9 (-159.4765, 481.419) -> (-159.4765, 460.419)
  arc A8 (-159.4765, 460.419) -> (-146.4765, 447.419) centre (-146.4765, 460.419) ccw
  line L10 (-146.4765, 447.419) -> (-86.4765, 447.419)
  arc A9 (-86.4765, 447.419) -> (-73.4765, 460.419) centre (-86.4765, 460.419) ccw
  line L11 (-73.4765, 460.419) -> (-73.4765, 481.419)
  circle A10 centre (-77.4765, 477.419) radius 20
  circle A11 centre (-155.4765, 477.419) radius 20
  circle A12 centre (-121.4765, 440.419) radius 16.7
  circle A13 centre (-111.4765, 440.419) radius 16.7
  line L12 (-140.4765, 459.419) -> (-146.4765, 459.419)
  arc A14 (-146.4765, 459.419) -> (-146.4765, 447.419) centre (-146.4765, 453.419) ccw
  line L13 (-146.4765, 447.419) -> (-140.4765, 447.419)
  arc A15 (-140.4765, 447.419) -> (-140.4765, 459.419) centre (-140.4765, 453.419) ccw
  line L14 (-140.4765, 453.419) -> (-146.4765, 453.419) construction
  line L15 (-92.4765, 447.419) -> (-86.4765, 447.419)
  arc A16 (-86.4765, 447.419) -> (-86.4765, 459.419) centre (-86.4765, 453.419) ccw
  line L16 (-86.4765, 459.419) -> (-92.4765, 459.419)
  arc A17 (-92.4765, 459.419) -> (-92.4765, 447.419) centre (-92.4765, 453.419) ccw
  line L17 (-92.4765, 453.419) -> (-86.4765, 453.419) construction
  line L18 (-106.4765, 459.119) -> (-126.4765, 459.119)
  line L19 (-134.4765, 467.119) -> (-134.4765, 469.719)
  line L20 (-126.4765, 477.719) -> (-106.4765, 477.719)
  line L21 (-98.4765, 469.719) -> (-98.4765, 467.119)
  arc A18 (-126.4765, 477.719) -> (-134.4765, 469.719) centre (-126.4765, 469.719) ccw
  arc A19 (-98.4765, 469.719) -> (-106.4765, 477.719) centre (-106.4765, 469.719) ccw
  arc A20 (-134.4765, 467.119) -> (-126.4765, 459.119) centre (-126.4765, 467.119) ccw
  arc A21 (-106.4765, 459.119) -> (-98.4765, 467.119) centre (-106.4765, 467.119) ccw
  circle A22 centre (-121.4765, 440.419) radius 1.7
  circle A23 centre (-116.5663, 496.419) radius 1.7
  circle A24 centre (-136.4765, 496.419) radius 1.7
  circle A25 centre (-96.4765, 496.419) radius 1.7
  circle A26 centre (-111.4765, 440.419) radius 1.7
  dimension "d116" = 12
  dimension "d117" = 12
  dimension "d123" = 6
  dimension "d124" = 6
  dimension "d125" = 6
  dimension "d126" = 6
  dimension "d128" = 8
  constraint horizontal L4
  constraint vertical L5
  constraint horizontal L6
  constraint vertical L7
  constraint tangent A1 L7
  constraint tangent A0 L5
  constraint tangent L12 A14
  constraint tangent A14 L13
  constraint parallel L12 L13
  constraint tangent L13 A15
  constraint tangent L12 A15
  constraint horizontal L14
  constraint coincident A8.end L10.start
  constraint tangent L15 A16
  constraint tangent A16 L16
  constraint parallel L15 L16
  constraint tangent L16 A17
  constraint tangent L15 A17
  constraint horizontal L17
  constraint coincident L10.end A9.start
  constraint parallel L6 L18
  constraint parallel L7 L19
  constraint parallel L4 L20
  constraint parallel L5 L21
  constraint tangent L19 A18
  constraint tangent L20 A18
  constraint tangent L20 A19
  constraint tangent L21 A19
  constraint equal A18 A19
  constraint tangent L18 A20
  constraint tangent L19 A20
  constraint equal A18 A20
  constraint tangent L18 A21
  constraint tangent L21 A21
  constraint equal A18 A21
  constraint concentric A3 A6
  constraint parallel L2 L8
  constraint concentric A4 A7
  constraint parallel L3 L9
  constraint concentric A5 A8
  constraint parallel L0 L10
  constraint concentric A2 A9
  constraint parallel L1 L11
  constraint tangent A6 L11
  constraint tangent A6 L8
  constraint tangent L10 A9
  constraint tangent A8 L10
  constraint tangent A7 L9
  constraint tangent L9 A8
  constraint tangent A9 L11
  measures "d123" radius of A14
  measures "d124" distance of A15.centre A14.centre
  measures "d125" radius of A17
  measures "d126" distance of A17.centre A16.centre
  measures "d128" radius of A18
extrude "Extrude9" cut sketch "Sketch3" against normal blind 6 contours L18 L19 L20 L21 A18 A19 A20 A21
fillet "Fillet1" radius 2 16 edges at (98.4765, 53.6943, 468.419) (100.8196, 53.6943, 475.3759) (116.4765, 53.6943, 477.719) (132.1333, 53.6943, 475.3759) (134.4765, 53.6943, 468.419) (132.1333, 53.6943, 461.4622) (116.4765, 53.6943, 459.119) (100.8196, 53.6943, 461.4622) (134.4765, 58.6943, 468.419) (132.1333, 58.6943, 475.3759) (116.4765, 58.6943, 477.719) (100.8196, 58.6943, 475.3759) (98.4765, 58.6943, 468.419) (100.8196, 58.6943, 461.4622) (116.4765, 58.6943, 459.119) (132.1333, 58.6943, 461.4622)
sketch "Sketch4" plane through (0, 53.6943, 0) normal (0, -1, 0) x (1, 0, 0)
  line L0 (86.4765, 435.419) -> (146.4765, 435.419)
  arc A0 (146.4765, 435.419) -> (171.4765, 460.419) centre (146.4765, 460.419) ccw
  line L1 (171.4765, 460.419) -> (171.4765, 481.419)
  arc A1 (171.4765, 481.419) -> (151.4765, 501.419) centre (151.4765, 481.419) ccw
  line L2 (151.4765, 501.419) -> (81.4765, 501.419)
  arc A2 (81.4765, 501.419) -> (61.4765, 481.419) centre (81.4765, 481.419) ccw
  line L3 (61.4765, 481.419) -> (61.4765, 460.419)
  arc A3 (61.4765, 460.419) -> (86.4765, 435.419) centre (86.4765, 460.419) ccw
  circle A4 centre (155.4765, 477.419) radius 8
  circle A5 centre (77.4765, 477.419) radius 8
  circle A6 centre (111.4765, 440.419) radius 1.7
  circle A7 centre (96.4765, 496.419) radius 1.7
  circle A8 centre (136.4765, 496.419) radius 1.7
  circle A9 centre (116.5663, 496.419) radius 1.7
  circle A10 centre (121.4765, 440.419) radius 1.7
  line L4 (96.4765, 467.119) -> (96.4765, 469.719)
  arc A11 (106.4765, 479.719) -> (96.4765, 469.719) centre (106.4765, 469.719) ccw
  line L5 (106.4765, 479.719) -> (126.4765, 479.719)
  arc A12 (136.4765, 469.719) -> (126.4765, 479.719) centre (126.4765, 469.719) ccw
  line L6 (136.4765, 469.719) -> (136.4765, 467.119)
  arc A13 (126.4765, 457.119) -> (136.4765, 467.119) centre (126.4765, 467.119) ccw
  line L7 (126.4765, 457.119) -> (106.4765, 457.119)
  arc A14 (96.4765, 467.119) -> (106.4765, 457.119) centre (106.4765, 467.119) ccw
  circle A15 centre (77.4765, 477.419) radius 9.5
  circle A16 centre (155.4765, 477.419) radius 9.5
  dimension "d133" = 19
  dimension "d134" = 19
  constraint concentric A5 A15
  constraint concentric A4 A16
  measures "d133" diameter of A15
  measures "d134" diameter of A16
extrude "Extrude10" cut sketch "Sketch4" against normal blind 1.1 contours A15 | A16
fillet "Fillet2" radius 0.4 6 edges at (146.6193, 53.6943, 480.8544) (158.3694, 54.7943, 469.9604) (158.3694, 58.6943, 469.9604) (80.3694, 58.6943, 469.9604) (80.3694, 54.7943, 469.9604) (68.6193, 53.6943, 480.8544)
extrude "Extrude3" [suppressed]
extrude "Extrude2" [suppressed]
extrude "Extrude4" [suppressed]
extrude "Extrude5" [suppressed]
extrude "Extrude6" [suppressed]
combine "Combine1" [suppressed]
equation "d3 = d2"
equation "d6 = d5 / 2"
equation "d33 = d32 / 2"
equation "d35 = d34 / 2"
equation "d125 = d123"
equation "d126 = d124"
equation "d134 = d133"
